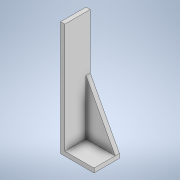
# Autodesk Inventor part: Mounting_ID6_Support
Saved by Autodesk Inventor 2022.2 (Build 262287010, 287A)
## iProperties
Created: 2024-09-30
Part Number: Mounting_ID6_Support
Material: Generisch
Document SubType Name: Modeling
Designer: ppovolni
Density: 1 g/cm^3
Appearance: Vorgabe
Author: ppovolni
Autodesk Inventor part; units mm, degrees
ref_plane "YZ Plane" through (0, 0, 0) normal (1, 0, 0) x (0, 1, 0)
ref_plane "XZ Plane" through (0, 0, 0) normal (0, 1, 0) x (-1, 0, 0)
ref_plane "XY Plane" through (0, 0, 0) normal (0, 0, 1) x (1, 0, 0)
sketch "Skizze1" plane through (0, 0, 0) normal (0, 0, 1) x (1, 0, 0)
  line L0 (0, 135) -> (0, 0)
  line L1 (0, 0) -> (39.478, 0)
  line L2 (39.478, 0) -> (39.478, 5)
  line L3 (39.478, 5) -> (5, 5)
  line L4 (5, 5) -> (5, 135)
  line L5 (5, 135) -> (0, 135)
  dimension "d0" = 39.478
  dimension "d1" = 5
  dimension "d2" = 135
  dimension "d5" = 5
  constraints: 12 end point, 4 perpendicular, 2 vertical
  measures "d0" distance of L0.end L1.end
  measures "d1" distance of L1.end L2.end
  measures "d2" distance of L0.start L0.end
  measures "d5" distance between parallel lines of L0 L4
extrude "Extrusion1" add sketch "Skizze1" along normal blind 30
sketch "Skizze2" plane through (0, 0, 0) normal (0, 0, -1) x (-1, 0, 0)
  line L0 (-5, 5) -> (-5, 135) projected
  line L1 (-39.478, 5) -> (-5, 5) projected
  line L2 (-39.478, 5) -> (-5, 70)
  point P0 (0, 0)
  constraints: 2 end point, 1 midpoint
extrude "Extrusion2" add sketch "Skizze2" against normal blind 5
